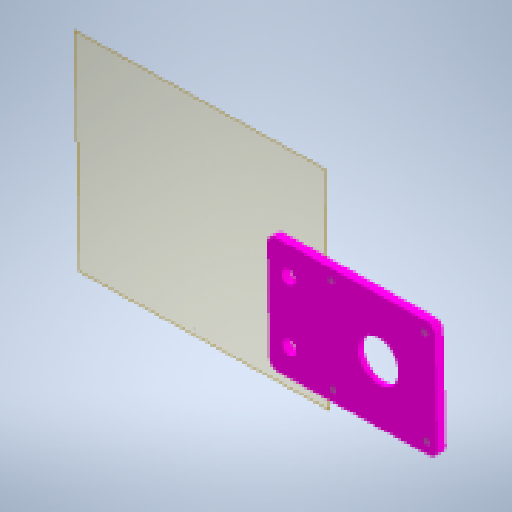
# Autodesk Inventor part: mocowanie silnika
Saved by Autodesk Inventor 2023 (Build 270158000, 158)
## iProperties
Created: 2023-04-14
Part Number: mocowanie silnika
Material: Tytan
Document SubType Name: Modeling
Designer: krzys
Density: 4.51 g/cm^3
Appearance: Fioletowe
Mass: 244.493 g
Surface Area: 235.377 cm^2
Volume: 54.2112 cm^3
Author: krzys
Autodesk Inventor part; units mm, degrees
ref_plane "YZ Plane" through (0, 0, 0) normal (1, 0, 0) x (0, 1, 0)
ref_plane "XZ Plane" through (0, 0, 0) normal (0, 1, 0) x (-1, 0, 0)
ref_plane "XY Plane" through (0, 0, 0) normal (0, 0, 1) x (1, 0, 0)
ref_plane "Płaszczyzna konstrukcyjna1" through (4579.4219, 19.0868, 0) normal (0, 0, 1) x (0.9997927, 0.0203617, 0)
sketch "Szkic1" plane through (4579.4219, 19.0868, 0) normal (0, 0, 1) x (0.9997927, 0.0203617, 0)
  circle A0 centre (85, 0) radius 5
  circle A1 centre (85, -45) radius 5
  line L0 (76, 21) -> (189, 21)
  line L1 (195, 15) -> (195, -59)
  line L2 (189, -65) -> (76, -65)
  line L3 (70, -59) -> (70, 15)
  arc A2 (70, -59) -> (76, -65) centre (76, -59) ccw
  arc A3 (76, 21) -> (70, 15) centre (76, 15) ccw
  arc A4 (189, -65) -> (195, -59) centre (189, -59) ccw
  arc A5 (195, 15) -> (189, 21) centre (189, 15) ccw
  circle A6 centre (152, -22) radius 30
  circle A7 centre (152, -22) radius 15
  line L4 (117.2, 12.8) -> (186.8, -56.8) construction
  line L5 (186.8, 12.8) -> (117.2, -56.8) construction
  circle A8 centre (117.2, 12.8) radius 2.4
  circle A9 centre (117.2, -56.8) radius 2.4
  circle A10 centre (186.8, -56.8) radius 2.4
  circle A11 centre (186.8, 12.8) radius 2.4
  point P0 (-4578.8611, 74.1621)
  point P1 (195, -65)
  point P2 (195, 21)
  point P3 (70, -65)
  dimension "d0" = 10
  dimension "d1" = 10
  dimension "d2" = 125
  dimension "d3" = 86
  dimension "d4" = 6
  dimension "d7" = 45
  dimension "d8" = 60
  dimension "d9" = 30
  dimension "d10" = 69.6
  dimension "d11" = 69.6
  dimension "d12" = 4.8
  dimension "d13" = 4.8
  dimension "d14" = 4.8
  dimension "d15" = 4.8
  constraints: 12 centre point, 12 end point, 8 point on circle, 8 tangent, 6 point on line, 5 coincident, 3 equal radius, 2 midpoint, 2 parallel, 1 horizontal, 1 perpendicular
  measures "d0" diameter of A0
  measures "d1" diameter of A1
  measures "d2" distance of point (195, -65) point (70, -65)
  measures "d3" distance of point (195, 21) point (195, -65)
  measures "d4" radius of A2
  measures "d7" distance of A1.centre A0.centre
  measures "d8" diameter of A6
  measures "d9" diameter of A7
  measures "d10" distance of L4.end L5.end
  measures "d11" distance of L5.start L4.end
  measures "d12" diameter of A8
  measures "d13" diameter of A9
  measures "d14" diameter of A10
  measures "d15" diameter of A11
extrude "Wyciągnięcie proste1" add sketch "Szkic1" along normal blind 6 contours L0 A5 L1 A4 L2 A2 L3 A3 | A6
extrude "Wyciągnięcie proste2" cut sketch "Szkic1" along normal blind 2 contours A6
thread "Gwint1" size "M6x1" class "6H" standard "ANSI Metric M Profile" full length
thread "Gwint2" size "M6x1" class "6H" standard "ANSI Metric M Profile" full length
thread "Gwint3" size "M6x1" class "6H" standard "ANSI Metric M Profile" full length
thread "Gwint4" size "M6x1" class "6H" standard "ANSI Metric M Profile" full length
